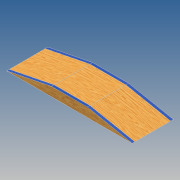
# Autodesk Inventor part: cad bestanden
Saved by Autodesk Inventor 2020 (Build 240168000, 168)
## iProperties
Created: 2019-11-19
Part Number: cad bestanden
Material: Generic
Document SubType Name: Modeling
Designer: Berkant
Density: 1 g/cm^3
Appearance: Default
Author: Berkant
Autodesk Inventor part; units mm, degrees
ref_plane "YZ Plane" through (0, 0, 0) normal (1, 0, 0) x (0, 1, 0)
ref_plane "XZ Plane" through (0, 0, 0) normal (0, 1, 0) x (-1, 0, 0)
ref_plane "XY Plane" through (0, 0, 0) normal (0, 0, 1) x (1, 0, 0)
sketch "Sketch1" plane through (0, 0, 0) normal (0, 0, 1) x (1, 0, 0)
  line L0 (0, 0) -> (400, 0)
  line L1 (400, 0) -> (400, 100)
  line L2 (400, 100) -> (0, 100)
  line L3 (0, 100) -> (0, 0)
  line L4 (400, 100) -> (451.0344, 100) construction
  line L5 (0, 100) -> (51.0344, 100) construction
  line L6 (400, 100) -> (900.4511, 0)
  line L7 (400, 100) -> (910.3443, 100) construction
  line L8 (900.4511, 0) -> (400, 0)
  line L9 (0, 100) -> (-500.4511, 0)
  line L10 (0, 100) -> (510.3443, 100) construction
  line L11 (-500.4511, 0) -> (0, 0)
  dimension "d0" = 400
  dimension "d1" = 100
  dimension "d6" = 11.3
  dimension "d7" = 168.7
  constraints: 24 end point, 6 horizontal, 2 equal length, 2 parallel, 2 perpendicular, 1 point on line
  measures "d0" distance of L2.end L1.end
  measures "d1" distance of L1.end L0.end
  measures "d6" angle of L6 L7
  measures "d7" angle of L9 L10
extrude "Extrusion1" add sketch "Sketch1" along normal blind 460
sketch "Sketch2" plane through (0, 100, 0) normal (0, 1, 0) x (1, 0, 0)
  line L0 (400, 0) -> (400, -460) projected
  line L1 (0, 0) -> (400, 0)
  line L2 (400, 0) -> (400, -30)
  line L3 (400, -30) -> (0, -30)
  line L4 (0, -30) -> (0, 0)
  line L5 (0, 0) -> (0, -460) projected
  line L6 (400, -460) -> (0, -460)
  line L7 (0, -460) -> (0, -430)
  line L8 (0, -430) -> (400, -430)
  line L9 (400, -430) -> (400, -460)
  dimension "d8" = 30
  dimension "d9" = 30
  constraints: 16 end point, 4 parallel, 2 horizontal, 2 perpendicular, 2 point on line
  measures "d8" distance of L1.end L2.end
  measures "d9" distance of L6.end L7.end
extrude "Extrusion2" add sketch "Sketch2" along normal blind 0.5 contours L0 L3 L4 L1 | L0 L6 L5 L8
sketch "Sketch3" plane through (900.4511, 0, 460) normal (0.1959, 0.9806, 0) x (0.9806, -0.1959, 0)
  line L0 (-1373.7453, 460) -> (0, 460) projected
  line L1 (-510.3443, 430) -> (-902.5902, 430) projected
  line L2 (0, 460) -> (-510.3443, 460)
  line L3 (-510.3443, 460) -> (-510.3443, 430)
  line L4 (-510.3443, 430) -> (0, 430)
  line L5 (0, 430) -> (0, 460)
  line L6 (0, 460) -> (0, 0) projected
  line L7 (-510.3443, 430) -> (-510.3443, 30) projected
  line L8 (0, 0) -> (-510.3443, 0)
  line L9 (-510.3443, 0) -> (-510.3443, 30)
  line L10 (-510.3443, 30) -> (0, 30)
  line L11 (0, 30) -> (0, 0)
  point P0 (-882.9956, 460)
  point P1 (-510.3443, 460)
  dimension "d12" = 30
  dimension "d13" = 510.3443
  dimension "d14" = 30
  constraints: 16 end point, 4 parallel, 2 horizontal, 2 perpendicular
  measures "d12" distance of L1.start L2.end
  measures "d13" distance of L7.end L10.end
  measures "d14" distance of L8.end L7.end
extrude "Extrusion3" add sketch "Sketch3" along normal blind 0.5 contours L0 L5 L4 L3 | L10 L6 L8 L9
sketch "Sketch4" plane through (-500.4511, 0, 460) normal (-0.1959, 0.9806, 0) x (0.9806, 0.1959, 0)
  line L0 (510.3443, 460) -> (0, 460) projected
  line L1 (902.5902, 430) -> (510.3443, 430) projected
  line L2 (0, 460) -> (510.3443, 460)
  line L3 (510.3443, 460) -> (510.3443, 430)
  line L4 (510.3443, 430) -> (0, 430)
  line L5 (0, 430) -> (0, 460)
  line L6 (510.3443, 0) -> (0, 0) projected
  line L7 (510.3443, 30) -> (902.5902, 30) projected
  line L8 (0, 0) -> (510.3443, 0)
  line L9 (510.3443, 0) -> (510.3443, 30)
  line L10 (510.3443, 30) -> (0, 30)
  line L11 (0, 30) -> (0, 0)
  point P0 (490.7497, 460)
  dimension "d17" = 30
  dimension "d18" = 30
  constraints: 16 end point, 4 parallel, 2 horizontal, 2 perpendicular
  measures "d17" distance of L2.end L1.end
  measures "d18" distance of L7.start L8.end
extrude "Extrusion4" add sketch "Sketch4" along normal blind 0.5
sketch "Sketch5" plane through (0, 0, 0) normal (0, 0, -1) x (-1, 0, 0)
  line L0 (0, 100.5) -> (-400, 100.5) projected
  line L1 (500.5491, 0.4903) -> (0.098, 100.4903) projected
  line L2 (0, 100.5) -> (0.098, 100.4903)
  line L3 (500.4511, 0) -> (0, 100) projected
  line L4 (0.098, 100.4903) -> (0, 100)
  line L5 (0, 100) -> (0, 100.5) projected
  line L6 (0, 100) -> (0, 100.5)
  point P0 (0, 0)
  constraints: 6 end point, 1 collinear, 1 perpendicular
extrude "Extrusion5" add sketch "Sketch5" against normal blind 460
sketch "Sketch6" plane through (0, 0, 0) normal (0, 0, -1) x (-1, 0, 0)
  line L0 (-400, 100) -> (-400, 100.5) projected
  line L1 (-400, 100.5) -> (-400, 100)
  line L2 (-400.098, 100.4903) -> (-900.5491, 0.4903) projected
  line L3 (-400, 100) -> (-400.098, 100.4903)
  line L4 (-400, 100.5) -> (0, 100.5) projected
  line L5 (-400.098, 100.4903) -> (-400, 100.5)
  point P0 (0, 0)
  constraints: 6 end point, 1 perpendicular, 1 vertical
extrude "Extrusion6" add sketch "Sketch6" against normal blind 460
body "Solid1"
